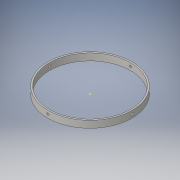
# Autodesk Inventor part: Sensing Gripper Crown
Saved by Autodesk Inventor 2016 (Build 200138000, 138)
## iProperties
Created: 2017-10-30
Part Number: Sensing Gripper Crown
Material: Generic
Document SubType Name: Modeling
Designer: ls769
Density: 1 g/cm^3
Appearance: Default
Author: ls769
Autodesk Inventor part; units mm, degrees
ref_plane "YZ Plane" through (0, 0, 0) normal (1, 0, 0) x (0, 1, 0)
ref_plane "XZ Plane" through (0, 0, 0) normal (0, 1, 0) x (-1, 0, 0)
ref_plane "XY Plane" through (0, 0, 0) normal (0, 0, 1) x (1, 0, 0)
sketch "Sketch1" plane through (0, 0, 0) normal (0, 1, 0) x (-1, 0, 0)
  circle A0 centre (0, 0) radius 41.073
  circle A1 centre (0, 0) radius 42.573
  dimension "d0" = 82.146
  dimension "d1" = 85.146
  constraints: 2 centre point, 1 coincident
  measures "d0" diameter of A0
  measures "d1" diameter of A1
extrude "Extrusion1" add sketch "Sketch1" along normal blind 7
sketch "Sketch2" plane through (0, 0, 0) normal (1, 0, 0) x (0, 1, 0)
  point P0 (0, 0)
sketch "Sketch3" plane through (0, 0, 0) normal (0, 0, 1) x (1, 0, 0)
  circle A0 centre (0, 3.5) radius 1.1
  point P0 (0, 0)
  dimension "d4" = 2.2
  constraints: 1 centre point
  measures "d4" diameter of A0
extrude "Extrusion2" cut sketch "Sketch3" along normal blind 57 and the other way blind 58.5
sketch "Sketch4" plane through (0, 0, 0) normal (1, 0, 0) x (0, 1, 0)
  circle A0 centre (3.5, 0) radius 1.1
  point P0 (0, 0)
  dimension "d9" = 2.2
  constraints: 1 centre point
  measures "d9" diameter of A0
extrude "Extrusion3" cut sketch "Sketch4" along normal blind 57 and the other way blind 58.5
body "Solid1"
